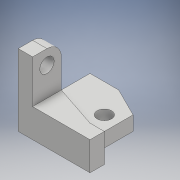
# Autodesk Inventor part: 30
Saved by Autodesk Inventor 2017 (Build 210142000, 142)
## iProperties
Part Number: 30
Material: 一般
Document SubType Name: Modeling
Designer: Brian
Density: 1 g/cm^3
Appearance: 預設
Author: Brian
Autodesk Inventor part; units mm, degrees
ref_plane "YZ Plane" through (0, 0, 0) normal (1, 0, 0) x (0, 1, 0)
ref_plane "XZ Plane" through (0, 0, 0) normal (0, 1, 0) x (-1, 0, 0)
ref_plane "XY Plane" through (0, 0, 0) normal (0, 0, 1) x (1, 0, 0)
sketch "草圖1" plane through (0, 0, 0) normal (0, 1, 0) x (-1, 0, 0)
  line L0 (0, 0) -> (-10, 0)
  line L1 (-10, 0) -> (-10, -50)
  line L2 (-10, -50) -> (0, -50)
  line L3 (0, -50) -> (0, 0)
  line L4 (-10, -50) -> (-50, -50)
  line L5 (-50, -50) -> (-50, -30)
  line L6 (-50, -30) -> (-10, -30)
  line L7 (-10, -30) -> (-10, -50)
  dimension "d0" = 20
  dimension "d1" = 10
  dimension "d2" = 50
  dimension "d3" = 40
  constraints: 16 end point, 4 parallel, 2 horizontal, 2 perpendicular
  measures "d0" distance of L4.end L5.end
  measures "d1" distance of L0.start L0.end
  measures "d2" distance of L0.end L1.end
  measures "d3" distance of L5.end L6.end
extrude "擠出1" add sketch "草圖1" along normal blind 20
sketch "草圖2" plane through (10, 0, -30) normal (0, 0, 1) x (1, 0, 0)
  line L0 (0, 0) -> (0, 20) projected
  line L1 (0, 20) -> (30, 10)
  line L2 (30, 10) -> (42.5125, 10)
  line L3 (0, 0) -> (40, 0) projected
  line L4 (0, 20) -> (41.4864, 29.1876)
  line L5 (41.4864, 29.1876) -> (42.5125, 10)
  point P0 (-10, 0)
  dimension "d6" = 10
  dimension "d7" = 30
  constraints: 8 end point, 1 perpendicular
  measures "d6" distance between parallel lines of L3 L2
  measures "d7" horizontal distance of L0.end L1.end
extrude "擠出2" cut sketch "草圖2" against normal through all
sketch "草圖3" plane through (50, 0, -50) normal (0, 0, -1) x (-1, 0, 0)
  line L0 (50, 0) -> (10, 0)
  line L1 (10, 0) -> (10, 50)
  line L2 (10, 50) -> (50, 50)
  line L3 (50, 50) -> (50, 0)
  dimension "d12" = 40
  dimension "d13" = 50
  constraints: 8 end point, 2 parallel, 1 horizontal, 1 perpendicular
  measures "d12" distance of L1.end L2.end
  measures "d13" distance of L0.end L1.end
extrude "擠出3" add sketch "草圖3" against normal blind 10
chamfer "倒角1" distance 10 distance2 20 1 edges at (40, 50, -45) measured on face at (40, 23.3333, -46.6667)
fillet "圓角1" radius 10 1 edges at (5, 20, 0)
sketch "草圖4" plane through (10, 0, 0) normal (1, 0, 0) x (0, 0, -1)
  circle A0 centre (10, 10) radius 5
  line L0 (0, 0) -> (30, 0) projected
  line L1 (0, 0) -> (0, 10) projected
  dimension "d20" = 10
  dimension "d21" = 10
  dimension "d22" = 10
  constraints: 1 centre point
  measures "d20" distance from line of L0 A0.centre
  measures "d21" distance from line of L1 A0.centre
  measures "d22" diameter of A0
extrude "擠出4" cut sketch "草圖4" against normal blind 10
sketch "草圖5" plane through (50, 0, -40) normal (0, 0, 1) x (1, 0, 0)
  circle A0 centre (-20, 30) radius 5
  line L0 (-10, 10) -> (-10, 40) projected
  point P0 (-50, 0)
  dimension "d25" = 10
  dimension "d26" = 10
  dimension "d27" = 10
  constraints: 1 centre point
  measures "d25" distance from line of L0 A0.centre
  measures "d26" horizontal distance of L0.end A0.centre
  measures "d27" diameter of A0
extrude "擠出5" cut sketch "草圖5" against normal blind 10
